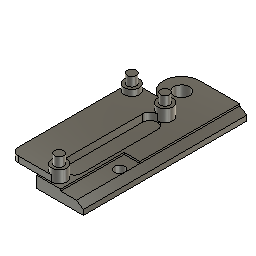
MotorMount (Autodesk Fusion 360 design; units mm, degrees)
Autodesk Fusion 360 part; units mm, degrees
note: some values were not read from the file. Set by a fixed rule: which face or edge a step refers to.
sketch "Sketch1" plane through (0, 0, 0) normal (0, 0, 1) x (1, 0, 0)
  circle A0 centre (0, 0) radius 1.3
  circle A1 centre (0, 0) radius 3
  line L0 (0, 0) -> (5.75, 0) construction
  line L1 (5.75, 0) -> (5.75, -16) construction
  line L2 (5.75, -16) -> (0, -16) construction
  line L3 (0, -16) -> (0, 0) construction
  circle A2 centre (5.75, -16) radius 0.85
  line L4 (0, 0) -> (0, -18)
  line L5 (0, -18) -> (7.75, -18)
  line L6 (7.75, -18) -> (7.75, 3)
  line L7 (7.75, 3) -> (0, 3)
  dimension "d1" = 2.6
  dimension "d2" = 6
  dimension "d3" = 5.75
  dimension "d4" = 16
  dimension "d5" = 1.7
  dimension "d6" = 18
  constraint coincident A0.centre A1.centre
  constraint concentric A0 A1
  constraint horizontal L0
  constraint vertical L1
  constraint horizontal L2
  constraint vertical L3
  constraint coincident L1.end L2.start
  constraint perpendicular L2 L4
  constraint perpendicular L4 L5
  constraint perpendicular L2 L6
  constraint coincident A1 L7.end
  constraint tangent A1 L7
  measures "d1" diameter of A0
  measures "d2" diameter of A1
  measures "d3" distance of A0.centre L0.end
  measures "d4" distance of A0.centre L2.end
  measures "d5" diameter of A2
  measures "d6" distance of A0.centre L4.end
extrude "Extrude1" add sketch "Sketch1" along normal blind 1.6
sketch "Sketch2" plane through (0, 0, 1.6) normal (0, 0, 1) x (-1, 0, 0)
  circle A0 centre (0, 0) radius 1.3
  circle A1 centre (-5.75, 16) radius 0.85
  line L0 (-7.75, -3) -> (0, -3)
  arc A2 (0, -3) -> (0, 3) centre (0, 0) ccw
  line L1 (0, 3) -> (0, 18)
  line L2 (0, 18) -> (-7.75, 18)
  line L3 (-7.75, 18) -> (-7.75, -3)
  circle A3 centre (0, 0) radius 3
  constraint coincident A0.centre A2.centre
  constraint coincident A2.end A3
extrude "Extrude2" add sketch "Sketch2" along normal blind 1.4 contours A2 A3
chamfer "Chamfer1" distance 1.15 distance2 0.75 1 edges at (7.75, -7.5, 1.6) measured on face at (1.709, -12.1406, 1.6)
sketch "Sketch3" plane through (0, 0, 1.6) normal (0, 0, 1) x (-1, 0, 0)
  line L0 (-6.6, 16) -> (-6.6, -3)
  line L1 (-6.6, -3) -> (0, -3)
  arc A0 (0, 3) -> (0, -3) centre (0, 0) ccw
  line L2 (0, 3) -> (0, 18)
  line L3 (0, 18) -> (-6.6, 18)
  line L4 (0, 18) -> (-4, 18)
  line L5 (-4, 18) -> (-4, -3)
  line L6 (-4, -3) -> (0, -3)
  line L7 (0, -3) -> (0, 18)
  line L8 (-4, 13.5) -> (-6.6, 13.5)
  line L9 (-7.75, -3) -> (-6.6, -3)
  line L10 (-6.6, -3) -> (0, -3)
  line L11 (-6.6, 13.5) -> (-6.6, -3)
  line L12 (-6.6, 18) -> (-6.6, 16)
  circle A1 centre (-5.75, 16) radius 0.85
  dimension "d13" = 21
  dimension "d16" = 2.6
  constraint horizontal L4
  constraint vertical L5
  constraint horizontal L6
  constraint vertical L7
  constraint coincident L2.end L3.start
  constraint horizontal L8
  constraint coincident L5 L8.start
  constraint coincident L9 L0.end
  constraint perpendicular L9 L11
  measures "d13" distance of L2.end L1.end
  measures "d16" distance of L8.start L8.end
extrude "Extrude3" add sketch "Sketch3" along normal blind 0.4 and the other way blind 0.5 contours L0 L1 L5 L8 L10 L11 | L1 A0 L2 L3 L4 L5 L6 L7 L10
move_face "OffsetFaces1" offset 4 3 faces at (6.1167, -18, 0.9) (2.6667, -18, 1.4333) (1.3333, -18, 1.7333)
sketch "Sketch4" plane through (0, 0, 2) normal (0, 0, 1) x (-1, 0, 0)
  line L0 (-4, 13.5) -> (-6.6, 13.5)
  line L1 (-6.6, 13.5) -> (-6.6, -3)
  line L2 (-6.6, -3) -> (0, -3)
  arc A0 (0, 3) -> (0, -3) centre (0, 0) ccw
  line L3 (0, 3) -> (0, 22)
  line L4 (0, 22) -> (-4, 22)
  line L5 (-4, 22) -> (-4, 13.5)
  line L6 (0, 0) -> (0, 5) construction
  line L7 (0, 5) -> (-2.25, 5)
  circle A1 centre (-2.25, 5) radius 1.25
  line L8 (-2.25, 5) -> (-2.25, 3.75) construction
  line L9 (-2.25, 3.75) -> (-2.25, 23.75) construction
  line L10 (-2.25, 23.75) -> (-2.25, 21.25) construction
  circle A2 centre (-2.25, 22.5) radius 1.25
  dimension "d20" = 5
  dimension "d21" = 2.25
  dimension "d22" = 2.5
  dimension "d23" = 20
  dimension "d24" = 2.5
  constraint coincident A0.centre L6.start
  constraint parallel L3 L6
  constraint perpendicular L3 L7
  constraint coincident L7.end A1.centre
  constraint coincident A1 L8.end
  constraint perpendicular L7 L8
  constraint perpendicular L7 L9
  constraint perpendicular L4 L10
  constraint coincident L10.end A2
  constraint coincident L9.end A2
  measures "d20" distance of A0.centre L6.end
  measures "d21" distance of L6.end L7.end
  measures "d22" diameter of A1
  measures "d23" distance of L8.end L9.end
  measures "d24" distance of L9.end L10.end
move_face "OffsetFaces2" offset 2 3 faces at (6.1167, -22, 0.9) (2.6667, -22, 1.4333) (1.3333, -22, 1.7333)
move_face "OffsetFaces3" offset 6 3 faces at (6.1167, -24, 0.9) (2.6667, -24, 1.4333) (1.3333, -24, 1.7333)
extrude "Extrude4" add sketch "Sketch4" along normal blind 1 contours L4 A2 | L4 A2 | A1
sketch "Sketch5" plane through (0, 0, 3) normal (0, 0, 1) x (-1, 0, 0)
  circle A0 centre (-2.25, 22.5) radius 1.25
  circle A1 centre (-2.25, 22.5) radius 0.75
  circle A2 centre (-2.25, 5) radius 1.25
  circle A3 centre (-2.25, 5) radius 0.75
  dimension "d29" = 1.5
  dimension "d30" = 1.5
  constraint concentric A0 A1
  constraint concentric A2 A3
  measures "d29" diameter of A1
  measures "d30" diameter of A3
extrude "Extrude5" add sketch "Sketch5" along normal blind 1 contours A1 | A3
sketch "Sketch6" plane through (0, 0, 2) normal (0, 0, 1) x (-1, 0, 0)
  circle A0 centre (-2.25, 5) radius 1.25
  circle A1 centre (-2.25, 22.5) radius 1.25
  line L0 (-4, 13.5) -> (-6.6, 13.5)
  line L1 (-6.6, 13.5) -> (-6.6, -3)
  line L2 (-6.6, -3) -> (0, -3)
  arc A2 (0, 3) -> (0, -3) centre (0, 0) ccw
  line L3 (0, 3) -> (0, 30)
  line L4 (0, 30) -> (-4, 30)
  line L5 (-4, 30) -> (-4, 13.5)
sketch "Sketch7" plane through (0, -30, 0) normal (0, -1, 0) x (1, 0, 0)
  line L0 (0, 2) -> (0, 0)
  line L1 (0, 0) -> (7.75, 0)
  line L2 (7.75, 0) -> (7.75, 0.85)
  line L3 (7.75, 0.85) -> (6.6, 1.6)
  line L4 (6.6, 1.6) -> (4, 1.6)
  line L5 (4, 1.6) -> (4, 2)
  line L6 (4, 2) -> (0, 2)
  line L7 (3.5, 3) -> (1, 3)
  line L8 (1, 2) -> (3.5, 2)
  line L9 (3.5, 2) -> (-3.5, 2)
  line L10 (-3.5, 2) -> (1, 2)
  line L11 (1, 2) -> (1, 6.5)
  line L12 (1, 6.5) -> (-3.5, 6.5)
  line L13 (-3.5, 6.5) -> (-3.5, 2)
  line L14 (1, 6.5) -> (-3.5, 2) construction
  circle A0 centre (-1.25, 4.25) radius 2.25
  line L15 (0, 2) -> (0, 2.3792)
  circle A1 centre (-1.25, 4.25) radius 3.25
  line L16 (-1.25, 4.25) -> (2, 4.25)
  line L17 (2, 4.25) -> (2, 2)
  line L18 (-3.5, 4.25) -> (-3, 0)
  line L19 (-3, 0) -> (-5.3, 0)
  line L20 (-3.5, 4.25) -> (-4.5, 4.25)
  line L21 (-4.5, 4.25) -> (-5.3, 0)
  dimension "d33" = 7
  dimension "d34" = 4.5
  dimension "d35" = 4.5
  dimension "d43" = 6.5
  constraint coincident L8.end L9.start
  constraint perpendicular L0 L9
  constraint horizontal L10
  constraint vertical L11
  constraint horizontal L12
  constraint vertical L13
  constraint tangent L10 A0
  constraint coincident L0.start L6.end
  constraint coincident A0 L15.end
  constraint perpendicular L10 L15
  constraint concentric A0 A1
  constraint coincident A0.centre A1.centre
  constraint coincident A1 L16.end
  constraint parallel L7 L16
  constraint midpoint L6 L17.end
  constraint midpoint L13 L18.start
  constraint parallel L16 L19
  constraint perpendicular L13 L20
  measures "d33" distance of L8.end L9.end
  measures "d34" distance of L9.end L8.start
  measures "d35" distance of L9.end L12.end
  measures "d43" diameter of A1
extrude "Extrude8" add sketch "Sketch7" against normal blind 4 from surface at -2 contours L6 L9 L10 L11 A0 L15 | L6 L7 L8 L9 L11 A1 | A1 L18 L19 L21 | L9 L10 L13 A1 L18 L20 | L6 L7 L8 L9 A1 L17 | L7 L11 A1 L16 | L9 L10 L13 A0 L18 | L11 L12 A0 | L11 L12 L13 A1 L16 L20 | L7 A1 L17 | L12 L13 A0
move_face "MoveFace1" by (0, 0, -0.1) 8 faces at (3.3333, -27.3333, 2) (0.3515, -22.9549, 2) (2.0833, -19.0833, 2) (1.8235, -12.4924, 2) (1.1713, -22.5621, 3) (2.0568, -22.6955, 4) (1.1741, -4.9006, 3) (2.2831, -5.1863, 4)
sketch "Sketch8" plane through (0, -30, 0) normal (0, -1, 0) x (1, 0, 0)
  line L0 (0, 1.9) -> (0, 0)
  line L1 (0, 0) -> (7.75, 0)
  line L2 (7.75, 0) -> (7.75, 0.85)
  line L3 (7.75, 0.85) -> (6.6, 1.6)
  line L4 (6.6, 1.6) -> (4, 1.6)
  line L5 (4, 1.6) -> (4, 1.9)
  line L6 (4, 1.9) -> (0, 1.9)
  line L7 (7.75, 0) -> (-5.3, 0)
  line L8 (-5.3, 0) -> (-5.3, 7.5)
  line L9 (-5.3, 7.5) -> (7.75, 7.5)
  line L10 (7.75, 7.5) -> (7.75, 0)
  constraint horizontal L7
  constraint vertical L8
  constraint horizontal L9
  constraint vertical L10
  constraint coincident L1.end L2.start
extrude "Extrude9" cut sketch "Sketch8" against normal blind 6
sketch "Sketch9" plane through (0, 0, 1.9) normal (0, 0, 1) x (-1, 0, 0)
  circle A0 centre (-2.25, 22.5) radius 1.25
  circle A1 centre (-2.25, 5) radius 1.25
  line L0 (0, 24) -> (-4, 24)
  line L1 (-4, 24) -> (-4, 13.5)
  line L2 (-4, 13.5) -> (-6.6, 13.5)
  line L3 (-6.6, 13.5) -> (-6.6, -3)
  line L4 (-6.6, -3) -> (0, -3)
  arc A2 (0, 3) -> (0, -3) centre (0, 0) ccw
  line L5 (0, 3) -> (0, 24)
  circle A3 centre (-2.25, 5) radius 1.25
  circle A4 centre (-2.25, 22.5) radius 1.25
  line L6 (-2.25, 22.5) -> (-2.25, 5) construction
  line L7 (-1, 6.25) -> (-3.5, 6.25)
  line L8 (-3.5, 6.25) -> (-3.5, 21.25)
  line L9 (-3.5, 21.25) -> (-1, 21.25)
  line L10 (-1, 21.25) -> (-1, 6.25)
  line L11 (-1, 6.25) -> (-3.5, 21.25) construction
  line L12 (-3.5, 6.25) -> (-1, 21.25) construction
  point P0 (-2.25, 13.75)
  dimension "d49" = 2.5
  dimension "d50" = 15
  constraint coincident A0.centre A4.centre
  constraint coincident A1.centre A3.centre
  constraint horizontal L7
  constraint perpendicular L7 L8
  constraint parallel L7 L9
  constraint parallel L8 L10
  constraint coincident L11 P0
  constraint coincident L12 P0
  constraint midpoint L6 P0
  measures "d49" distance of L8.end L9.end
  measures "d50" distance of L7.end L8.end
extrude "Extrude10" cut sketch "Sketch9" against normal blind 0.2 contours L7 L8 L9 L10
fillet "Fillet1" radius 1.25 4 edges at (1, -6.25, 1.8) (3.5, -6.25, 1.8) (3.5, -21.25, 1.8) (1, -21.25, 1.8)
sketch "Sketch10" plane through (0, 0, 3) normal (0, 0, 1) x (-1, 0, 0)
  circle A0 centre (0, 0) radius 1.3
  circle A1 centre (0, 0) radius 3
extrude "Extrude11" cut sketch "Sketch10" against normal blind 1.1
sketch "Sketch11" plane through (0, 0, 1.9) normal (0, 0, 1) x (-1, 0, 0)
  circle A0 centre (0, 0) radius 1.3
  line L0 (0, 24) -> (-4, 24)
  line L1 (-4, 24) -> (-4, 13.5)
  line L2 (-4, 13.5) -> (-6.6, 13.5)
  line L3 (-6.6, 13.5) -> (-6.6, -3)
  line L4 (-6.6, -3) -> (0, -3)
  arc A1 (0, -3) -> (0, 3) centre (0, 0) ccw
  line L5 (0, 3) -> (0, 24)
  circle A2 centre (-2.25, 5) radius 1.25
  arc A3 (-3.5, 7.5) -> (-2.25, 6.25) centre (-2.25, 7.5) ccw
  line L6 (-3.5, 7.5) -> (-3.5, 20)
  arc A4 (-2.25, 21.25) -> (-3.5, 20) centre (-2.25, 20) ccw
  circle A5 centre (-2.25, 22.5) radius 1.25
  arc A6 (-1, 20) -> (-2.25, 21.25) centre (-2.25, 20) ccw
  line L7 (-1, 20) -> (-1, 7.5)
  arc A7 (-2.25, 6.25) -> (-1, 7.5) centre (-2.25, 7.5) ccw
  line L8 (-2.25, 5) -> (-3.5, 5) construction
  line L9 (-3.5, 5) -> (-3.5, 3.75) construction
  line L10 (-3.5, 3.75) -> (-2.25, 3.75) construction
  line L11 (-2.25, 3.75) -> (-2.25, 5) construction
  line L12 (-3.5, 3.75) -> (3.25, 3.75)
  line L13 (4.5, 5) -> (4.5, 22.5)
  line L14 (3.25, 23.75) -> (-3.5, 23.75)
  line L15 (-3.5, 23.75) -> (-3.5, 3.75)
  arc A8 (3.25, 3.75) -> (4.5, 5) centre (3.25, 5) ccw
  arc A9 (4.5, 22.5) -> (3.25, 23.75) centre (3.25, 22.5) ccw
  point P0 (4.5, 3.75)
  dimension "d57" = 1.25
  dimension "d58" = 1.25
  dimension "d59" = 8
  dimension "d60" = 20
  dimension "d61" = 1.25
  dimension "d62" = 1.25
  constraint horizontal L8
  constraint vertical L9
  constraint horizontal L10
  constraint vertical L11
  constraint coincident A2.centre L8.start
  constraint horizontal L12
  constraint vertical L13
  constraint horizontal L14
  constraint vertical L15
  constraint coincident P0 L12
  constraint coincident P0 L13
  constraint tangent L12 A8
  constraint tangent L13 A8
  constraint tangent L13 A9
  constraint tangent L14 A9
  measures "d57" distance of A2.centre L8.end
  measures "d58" distance of A2.centre L10.end
  measures "d59" distance of L9.end P0
  measures "d60" distance of L9.end L14.end
  measures "d61" radius of A8
  measures "d62" radius of A9
move_face "MoveFace2" by (0, 0, 1) 4 faces at (2.2831, -5.1863, 3.9) (1.1741, -4.9006, 2.9) (2.0568, -22.6955, 3.9) (1.1713, -22.5621, 2.9)
extrude "Extrude12" add sketch "Sketch11" along normal blind 1 contours L5 L12 L13 L14 A8 A9 | L5 A2 A5 A6 L7 A7 L12 L14
sketch "Sketch12" plane through (0, 0, 2.9) normal (0, 0, 1) x (-1, 0, 0)
  line L0 (-2.25, 3.75) -> (3.25, 3.75)
  arc A0 (3.25, 3.75) -> (4.5, 5) centre (3.25, 5) ccw
  line L1 (4.5, 5) -> (4.5, 22.5)
  arc A1 (4.5, 22.5) -> (3.25, 23.75) centre (3.25, 22.5) ccw
  line L2 (3.25, 23.75) -> (-2.25, 23.75)
  arc A2 (-2.25, 21.25) -> (-2.25, 23.75) centre (-2.25, 22.5) ccw
  arc A3 (-1, 20) -> (-2.25, 21.25) centre (-2.25, 20) ccw
  line L3 (-1, 20) -> (-1, 7.5)
  arc A4 (-2.25, 6.25) -> (-1, 7.5) centre (-2.25, 7.5) ccw
  arc A5 (-2.25, 3.75) -> (-2.25, 6.25) centre (-2.25, 5) ccw
  circle A6 centre (3.25, 5) radius 1.25
  constraint concentric A0 A6
  constraint coincident L0.end A6
extrude "Extrude13" add sketch "Sketch12" along normal blind 1 contours A0 A6
move_face "MoveFace3" by (0, 0, 0.5) 2 faces at (2.2831, -5.1863, 4.9) (2.0568, -22.6955, 4.9)
sketch "Sketch13" plane through (0, 0, 3.9) normal (0, 0, 1) x (-1, 0, 0)
  circle A0 centre (3.25, 5) radius 1.25
  circle A1 centre (3.25, 5) radius 0.75
  dimension "d67" = 1.5
  constraint concentric A0 A1
  measures "d67" diameter of A1
extrude "Extrude14" add sketch "Sketch13" along normal blind 1.5 contours A1
